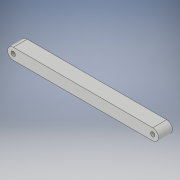
# Autodesk Inventor part: Lever
Saved by Autodesk Inventor 2019.1 (Build 231200000, 200)
## iProperties
Created: 2018-11-01
Part Number: Lever
Material: Generisch
Document SubType Name: Modeling
Designer: JochenAlt
Density: 1 g/cm^3
Appearance: Vorgabe
Author: JochenAlt
Autodesk Inventor part; units mm, degrees
ref_plane "YZ Plane" through (0, 0, 0) normal (1, 0, 0) x (0, 1, 0)
ref_plane "XZ Plane" through (0, 0, 0) normal (0, 1, 0) x (-1, 0, 0)
ref_plane "XY Plane" through (0, 0, 0) normal (0, 0, 1) x (1, 0, 0)
sketch "Skizze1" plane through (0, 0, 0) normal (0, 0, 1) x (1, 0, 0)
  line L0 (0, 0) -> (80, 0) construction
  line L1 (0, -3.25) -> (80, -3.25)
  line L2 (80, 3.25) -> (0, 3.25)
  arc A0 (0, 3.25) -> (0, -3.25) centre (0, 0) ccw
  arc A1 (80, -3.25) -> (80, 3.25) centre (80, 0) ccw
  circle A2 centre (0, 0) radius 1.25
  circle A3 centre (80, 0) radius 1.25
  point P0 (40, 0)
  dimension "d0" = 2.5
  dimension "d1" = 2
  dimension "d2" = 80
  constraints: 8 end point, 4 centre point, 4 point on circle, 4 tangent, 2 coincident, 1 equal radius, 1 horizontal, 1 midpoint, 1 parallel
  measures "d0" diameter of A2
  measures "d1" radial gap between concentric circles of A0 A2
  measures "d2" distance of L0.end L0.start
extrude "Extrusion1" add sketch "Skizze1" along normal blind 8
